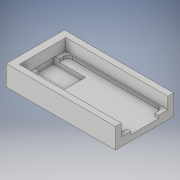
# Autodesk Inventor part: PiHolder
Saved by Autodesk Inventor 2019 (Build 230136000, 136)
## iProperties
Created: 2019-04-12
Part Number: PiHolder
Material: Generic
Document SubType Name: Modeling
Designer: Epsilon
Density: 1 g/cm^3
Appearance: Default
Author: Epsilon
Autodesk Inventor part; units mm, degrees
ref_plane "YZ Plane" through (0, 0, 0) normal (1, 0, 0) x (0, 1, 0)
ref_plane "XZ Plane" through (0, 0, 0) normal (0, 1, 0) x (-1, 0, 0)
ref_plane "XY Plane" through (0, 0, 0) normal (0, 0, 1) x (1, 0, 0)
sketch "Sketch2" plane through (0, 0, 0) normal (0, 1, 0) x (-1, 0, 0)
  line L0 (0, 0) -> (75, 0)
  line L1 (75, 0) -> (75, -40)
  line L2 (75, -40) -> (0, -40)
  line L3 (0, -40) -> (0, 0)
  dimension "d4" = 75
  dimension "d5" = 40
  constraints: 8 end point, 2 parallel, 1 horizontal, 1 perpendicular
  measures "d4" distance of L1.end L2.end
  measures "d5" distance of L0.end L1.end
extrude "Extrusion2" add sketch "Sketch2" along normal blind 14
sketch "Sketch4" plane through (0, 14, 0) normal (0, 1, 0) x (1, 0, 0)
  line L0 (0, 0) -> (0, 40) projected
  line L1 (0, 4) -> (-70, 4)
  line L2 (-70, 4) -> (-70, 36)
  line L3 (-70, 36) -> (0, 36)
  line L4 (0, 36) -> (0, 4)
  line L5 (-75, 40) -> (-75, 0) construction
  line L6 (-75, 20) -> (0, 20) construction
  dimension "d8" = 70
  dimension "d9" = 32
  constraints: 10 end point, 2 midpoint, 2 parallel, 2 perpendicular, 1 horizontal, 1 point on line, 1 other
  measures "d8" distance of L2.end L3.end
  measures "d9" distance of L1.end L2.end
extrude "Extrusion3" cut sketch "Sketch4" against normal blind 10
sketch "Sketch5" plane through (0, 4, 0) normal (0, 1, 0) x (1, 0, 0)
  line L0 (0, 4) -> (-70, 4) projected
  line L1 (-70, 36) -> (0, 36) projected
  line L2 (0, 4) -> (-70, 4)
  line L3 (-70, 4) -> (-70, 36)
  line L4 (-70, 36) -> (0, 36)
  line L5 (0, 36) -> (0, 10.475)
  line L6 (-2.5, 5) -> (-67.5, 5)
  line L7 (-67.5, 5) -> (-67.5, 35)
  line L8 (-67.5, 35) -> (-2.5, 35)
  line L9 (-2.5, 35) -> (-2.5, 29.525)
  line L10 (0, 40) -> (0, 0) construction
  line L11 (0, 20) -> (-70, 20) construction
  line L12 (-70, 4) -> (-70, 36) construction
  line L13 (-35, 4) -> (-35, 35) construction
  line L14 (0, 36) -> (0, 4) projected
  line L15 (-2.5, 10.475) -> (0, 10.475)
  line L16 (0, 29.525) -> (-2.5, 29.525)
  line L17 (-2.5, 10.475) -> (-2.5, 5)
  line L18 (0, 10.475) -> (0, 4)
  dimension "d12" = 65
  dimension "d13" = 30
  dimension "d17" = 19.05
  constraints: 28 end point, 7 parallel, 4 midpoint, 3 horizontal, 3 perpendicular, 1 point on line, 4 other
  measures "d12" distance of L7.end L8.end
  measures "d13" distance of L6.end L7.end
  measures "d17" distance of L16.start L5.end
extrude "Extrusion5" add sketch "Sketch5" along normal blind 2 contours L0 L3 L1 L5 L16 L9 L8 L7 L6 L17 L15 L14
fillet "Fillet2" radius 3 4 edges at (-2.5, 5, -5) (-67.5, 5, -5) (-67.5, 5, -35) (-2.5, 5, -35)
sketch "Sketch6" plane through (0, 4, 0) normal (0, 1, 0) x (1, 0, 0)
  line L0 (-67.5, 32) -> (-67.5, 8) projected
  line L1 (-67.5, 28.9) -> (-49.5, 28.9) construction
  line L2 (-49.5, 28.9) -> (-49.5, 14.9) construction
  line L3 (-49.5, 14.9) -> (-67.5, 14.9) construction
  line L4 (-67.5, 14.9) -> (-67.5, 28.9) construction
  line L5 (-67.5, 21.9) -> (-49.5, 21.9) construction
  line L6 (-5.5, 5) -> (-64.5, 5) construction
  line L7 (-67.5, 28.9) -> (-71.5, 28.9) construction
  line L8 (-71.5, 28.9) -> (-71.5, 14.9) construction
  line L9 (-71.5, 14.9) -> (-67.5, 14.9) construction
  line L10 (-67.5, 14.9) -> (-67.5, 28.9) construction
  line L11 (-71.5, 28.9) -> (-49.5, 28.9)
  line L12 (-49.5, 28.9) -> (-49.5, 14.9)
  line L13 (-49.5, 14.9) -> (-71.5, 14.9)
  line L14 (-71.5, 14.9) -> (-71.5, 28.9)
  point P0 (0, 0)
  dimension "d21" = 18
  dimension "d22" = 14
  dimension "d23" = 16.9
  dimension "d24" = 4
  constraints: 26 end point, 6 parallel, 3 horizontal, 3 perpendicular, 2 midpoint, 1 point on line
  measures "d21" distance of L2.end L3.end
  measures "d22" distance of L1.end L2.end
  measures "d23" distance between parallel lines of L6 L5
  measures "d24" distance of L9.end L8.end
extrude "Extrusion6" cut sketch "Sketch6" against normal blind 3 and the other way blind 2.54
body "Solid2"
